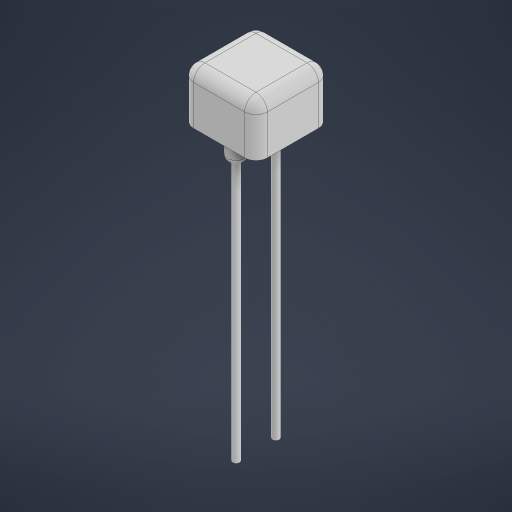
# Autodesk Inventor part: Part2
Saved by Autodesk Inventor 2024 (Build 280153000, 153)
## iProperties
Created: 2023-12-19
Part Number: Part2
Material: Generic
Document SubType Name: Sheet Metal
Designer: Shado
Density: 1 g/cm^3
Sheet Metal Rule: Default
Appearance: Default
Author: Shado
Autodesk Inventor part; units mm, degrees
ref_plane "YZ Plane" through (0, 0, 0) normal (1, 0, 0) x (0, 1, 0)
ref_plane "XZ Plane" through (0, 0, 0) normal (0, 1, 0) x (-1, 0, 0)
ref_plane "XY Plane" through (0, 0, 0) normal (0, 0, 1) x (1, 0, 0)
sketch "Sketch1" plane through (0, 0, 0) normal (0, 1, 0) x (-1, 0, 0)
  line L0 (1, 0) -> (5.5, 0)
  line L1 (6.5, -1) -> (6.5, -5.5)
  line L2 (5.5, -6.5) -> (1, -6.5)
  line L3 (0, -5.5) -> (0, -1)
  arc A0 (6.5, -1) -> (5.5, 0) centre (5.5, -1) ccw
  arc A1 (0, -5.5) -> (1, -6.5) centre (1, -5.5) ccw
  arc A2 (5.5, -6.5) -> (6.5, -5.5) centre (5.5, -5.5) ccw
  arc A3 (1, 0) -> (0, -1) centre (1, -1) ccw
  circle A4 centre (3.25, -5) radius 0.75
  circle A5 centre (3.25, -1.5) radius 0.75
  point P0 (0, 0)
  point P1 (6.5, -6.5)
  point P2 (6.5, 0)
  point P3 (0, -6.5)
  dimension "d0" = 6.5
  dimension "d1" = 6.5
  dimension "d2" = 1
  dimension "d5" = 1.5
  dimension "d7" = 1.5
  constraints: 8 end point, 8 point on circle, 8 point on line, 8 tangent, 6 centre point, 3 equal radius, 2 parallel, 1 horizontal, 1 perpendicular
  measures "d0" distance of point (6.5, -6.5) point (0, -6.5)
  measures "d1" distance of point (6.5, 0) point (6.5, -6.5)
  measures "d2" radius of A0
  measures "d5" diameter of A4
  measures "d7" diameter of A5
extrude "Extrusion1" add sketch "Sketch1" along normal blind 4.5 contours L0 A0 L1 A2 L2 A1 L3 A3 | A4 | A5
fillet "Fillet1" radius 1 8 edges at (-0.2929, 4.5, -6.2071) (-3.25, 4.5, -6.5) (-6.2071, 4.5, -6.2071) (-6.5, 4.5, -3.25) (-6.2071, 4.5, -0.2929) (-3.25, 4.5, 0) (-0.2929, 4.5, -0.2929) (0, 4.5, -3.25)
sketch "Sketch2" plane through (0, 0, 0) normal (0, -1, 0) x (1, 0, 0)
  circle A0 centre (-3.25, -1.5) radius 0.75
  circle A1 centre (-3.25, -5) radius 0.75
  point P0 (0, 0)
  dimension "d13" = 1.5
  dimension "d14" = 1.5
  constraints: 2 centre point
  measures "d13" diameter of A0
  measures "d14" diameter of A1
extrude "Extrusion2" add sketch "Sketch2" along normal blind 2
sketch "Sketch3" plane through (-3.25, -2, -1.5) normal (0, -1, 0) x (1, 0, 0)
  circle A0 centre (0, 0) radius 0.3
  circle A1 centre (0, -3.5) radius 0.75 projected
  circle A2 centre (0, -3.5) radius 0.3
  point P0 (3.25, 1.5)
  dimension "d17" = 0.6
  dimension "d18" = 0.6
  constraints: 2 centre point, 1 coincident
  measures "d17" diameter of A0
  measures "d18" diameter of A2
extrude "Extrusion3" add sketch "Sketch3" along normal blind 23 contours A0 | A2
fillet "Fillet2" radius 0.45 2 edges at (-4, -2, -1.5) (-4, -2, -5)
equation "\"BendRadius\" = Thickness"
equation "\"BendReliefWidth\" = Thickness"
equation "\"BendReliefDepth\" = 0.5 * Thickness"
equation "\"CornerReliefSize\" = 4 * Thickness"
equation "\"MinimumRemnant\" = 2 * Thickness"
equation "\"TransitionRadius\" = BendRadius"
equation "\"JacobiRadiusSize\" = BendRadius"
equation "\"GapSize\" = Thickness"
equation "\"Thickness\" = 3.048"
body "Solid1"
